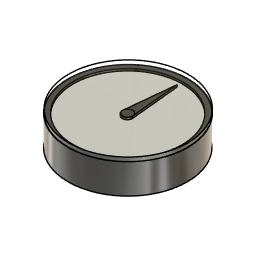
B.E.E.R. Compass Shell (Autodesk Fusion 360 design; units mm, degrees)
part number: 2025-05-31-00-10-06-116
Autodesk Fusion 360 part; units mm, degrees
cylinder "CylinderPrimitive1" add diameter 60 height 15 placed x (1, 0, 0) y (0, 1, 0) z (0, 0, 1) at (50, 50, 0) makes body 1
hole "Hole1" at (50, 50, 15) direction (0, 0, -1) diameter 55 depth 20 tip angle 118 bodies 1
cylinder "CylinderPrimitive2" add diameter 55 height 2 placed x (1, 0, 0) y (0, 1, 0) z (0, 0, 1) at (50, 50, 0) bodies 1
cylinder "CylinderPrimitive3" add diameter 60 height 2 placed x (1, 0, 0) y (0, 1, 0) z (0, 0, 1) at (-75, 75, 0) separate body makes body 2
move_body "Move1" bodies 2 to x (1, 0, 0) y (0, 1, 0) z (0, 0, 1) at (125.1699, -25.1206, 15)
move_body "Move2" bodies 2 to x (1, 0, 0) y (0, 1, 0) z (0, 0, 1) at (88.8366, 2.8621, 14.9088)
cylinder "CylinderPrimitive4" add diameter 55 height 1 placed x (1, 0, 0) y (0, 1, 0) z (0, 0, 1) at (-100, 60, 0) separate body makes body 3
move_body "Move3" bodies 3 to x (1, 0, 0) y (0, 1, 0) z (0, 0, 1) at (0, 0, 13)
cylinder "CylinderPrimitive5" add diameter 5 height 15 placed x (1, 0, 0) y (0, 1, 0) z (0, 0, 1) at (-40, 50, 0) separate body makes body 4
move_body "Move4" bodies 4 to x (1, 0, 0) y (0, 1, 0) z (0, 0, 1) at (90, 0, 0)
move_body "Move5" bodies 3 to x (1, 0, 0) y (0, 1, 0) z (0, 0, 1) at (150, -10, 0)
move_body "Move6" bodies 2 to x (1, 0, 0) y (0, 1, 0) z (0, 0, 1) at (-89, -2.5, -15)
move_body "Move7" bodies 2 to x (1, 0, 0) y (0, 1, 0) z (0, 0, 1) at (-115, 0, 0)
sketch "Sketch7" plane through (0, 0, 0) normal (0, 0, 1) x (1, 0, 0)
  line L0 (50, 0) -> (74.9696, 2.4698)
  line L1 (74.9696, 2.4698) -> (50, 5)
  arc A0 (50, 5) -> (50, 0) centre (49.7467, 2.5) ccw
  constraint tangent L1 A0
extrude "Extrude1" add sketch "Sketch7" along normal blind 1 separate body makes body 5
move_body "Move8" bodies 5 to x (1, 0, 0) y (0, 1, 0) z (0, 0, 1) at (0, 0, 14)
move_body "Move9" bodies 5 to x (1, 0, 0) y (0, 1, 0) z (0, 0, 1) at (0, 47.5, 0)
move_body "Move10" bodies 5 to x (0, 1, 0) y (-1, 0, 0) z (0, 0, 1) at (100, 0, 0)
move_body "Move11" bodies 2 to x (1, 0, 0) y (0, 1, 0) z (0, 0, 1) at (115, 0, 0)
move_body "Move12" bodies 2 to x (1, 0, 0) y (0, 1, 0) z (0, 0, 1) at (-85, 0, 0)
move_body "Move13" bodies 2 to x (1, 0, 0) y (0, 1, 0) z (0, 0, 1) at (85, 0, 0)
